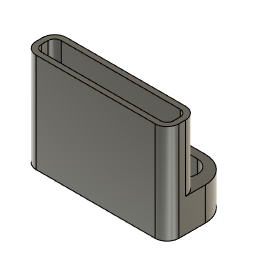
NG_4_CAD (Autodesk Fusion 360 design; units mm, degrees)
Autodesk Fusion 360 part; units mm, degrees
sketch "Sketch1" plane through (0, 0, 0) normal (0, 0, 1) x (1, 0, 0)
  line L0 (2, 0) -> (38, 0)
  line L1 (40, 2) -> (40, 4)
  line L2 (38, 6) -> (2, 6)
  line L3 (0, 4) -> (0, 2)
  arc A0 (2, 6) -> (0, 4) centre (2, 4) ccw
  arc A1 (0, 2) -> (2, 0) centre (2, 2) ccw
  arc A2 (38, 0) -> (40, 2) centre (38, 2) ccw
  arc A3 (40, 4) -> (38, 6) centre (38, 4) ccw
  line L4 (-1.6, 4) -> (-1.6, 2)
  arc A4 (-1.6, 2) -> (2, -1.6) centre (2, 2) ccw
  line L5 (2, -1.6) -> (38, -1.6)
  arc A5 (38, -1.6) -> (41.6, 2) centre (38, 2) ccw
  line L6 (41.6, 2) -> (41.6, 4)
  arc A6 (41.6, 4) -> (38, 7.6) centre (38, 4) ccw
  line L7 (38, 7.6) -> (2, 7.6)
  arc A7 (2, 7.6) -> (-1.6, 4) centre (2, 4) ccw
  line L8 (6.4, 15.6) -> (15.8, 15.6)
  arc A8 (6.4, 15.6) -> (6.4, 7.6) centre (6.4, 11.6) ccw
  line L9 (15.8, 18) -> (6.4, 18)
  line L10 (-1.6, 4) -> (-1.6, 10)
  arc A9 (6.4, 18) -> (-1.6, 10) centre (6.4, 10) ccw
  arc A10 (15.8, 15.6) -> (15.8, 18) centre (15.8, 16.8) ccw
  line L11 (20, 6) -> (20, 12.2133) construction
  arc A11 (33.6, 7.6) -> (33.6, 15.6) centre (33.6, 11.6) ccw
  line L12 (33.6, 15.6) -> (24.2, 15.6)
  line L13 (24.2, 18) -> (33.6, 18)
  arc A12 (24.2, 18) -> (24.2, 15.6) centre (24.2, 16.8) ccw
  arc A13 (41.6, 10) -> (33.6, 18) centre (33.6, 10) ccw
  line L14 (41.6, 4) -> (41.6, 10)
  line L15 (6.4, 10) -> (6.4, 11.6) construction
  line L16 (23, 16.8) -> (17, 16.8) construction
  point P0 (0, 6)
  dimension "d1" = 6
  dimension "d2" = 2
  dimension "d3" = 1.6
  dimension "d5" = 8
  dimension "d7" = 2.4
  dimension "d14" = 40
  dimension "d15" = 8
  dimension "d16" = 6
  constraint horizontal L0
  constraint vertical L1
  constraint horizontal L2
  constraint vertical L3
  constraint coincident P0 L2
  constraint coincident P0 L3
  constraint tangent L2 A0
  constraint tangent L3 A0
  constraint coincident origin L3
  constraint coincident origin L0
  constraint tangent L3 A1
  constraint tangent L0 A1
  constraint equal A0 A1
  constraint tangent L0 A2
  constraint tangent L1 A2
  constraint equal A0 A2
  constraint tangent L1 A3
  constraint tangent L2 A3
  constraint equal A0 A3
  constraint horizontal L8
  constraint coincident L7 A8.end
  constraint tangent L8 A8
  constraint horizontal L9
  constraint tangent A7 L10
  constraint parallel L4 L10
  constraint tangent L10 A9
  constraint tangent L7 A8
  constraint tangent L8 A10
  constraint midpoint L2 L11.start
  constraint perpendicular L2 L11
  constraint symmetric L4.start L11 L6.end
  constraint symmetric L8.start L11 A11.end
  constraint symmetric L8.end L11 L12.end
  constraint symmetric A8.end L11 A11.start
  constraint symmetric A8 L11 A11
  constraint symmetric L9.start L11 L13.start
  constraint symmetric L9.end L11 L13.end
  constraint symmetric L10.end L11 A13.start
  constraint symmetric A9 L11 A13
  constraint symmetric A10 L11 A12
  constraint tangent L9 A10
  constraint tangent L9 A9
  constraint coincident A9.centre L15.start
  constraint coincident A8.centre L15.end
  constraint vertical L15
  constraint midpoint A12 L16.start
  constraint midpoint A10 L16.end
  measures "d1" distance of origin P0
  measures "d2" radius of A0
  measures "d5" distance of L7 L8
  measures "d7" distance of L8 L9
  measures "d14" distance of L1 L3
  measures "d15" horizontal distance of A8.centre L10.end
  measures "d16" distance of L16.start L16.end
extrude "Extrude1" add sketch "Sketch1" along normal blind 10
extrude "Extrude2" add sketch "Sketch1" along normal blind 20 from surface at 10 contours L4 A4 L5 A5 L6 A6 L7 A7
